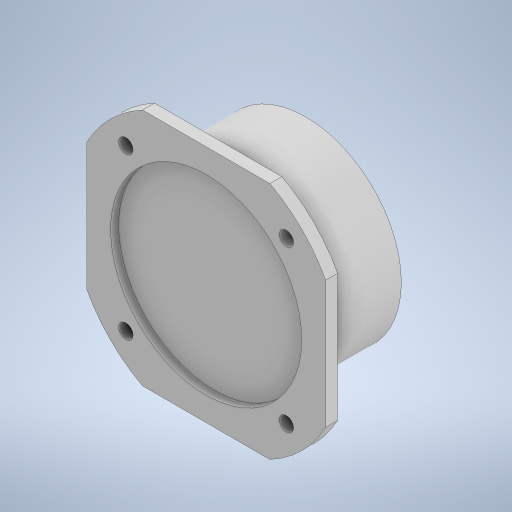
# Autodesk Inventor part: tweetwe
Saved by Autodesk Inventor 2023 (Build 270158000, 158)
## iProperties
Created: 2022-07-14
Part Number: tweetwe
Material: Generic
Document SubType Name: Modeling
Designer: Zain Ali
Density: 1 g/cm^3
Appearance: Default
Author: Zain Ali
Autodesk Inventor part; units mm, degrees
ref_plane "YZ Plane" through (0, 0, 0) normal (1, 0, 0) x (0, 1, 0)
ref_plane "XZ Plane" through (0, 0, 0) normal (0, 1, 0) x (-1, 0, 0)
ref_plane "XY Plane" through (0, 0, 0) normal (0, 0, 1) x (1, 0, 0)
sketch "Sketch1" plane through (0, 0, 0) normal (0, 0, 1) x (1, 0, 0)
  circle A0 centre (0, 0) radius 23.5 construction
  circle A1 centre (0, 0) radius 34 construction
  line L0 (30, 30) -> (-30, 30) construction
  line L1 (-30, 30) -> (-30, -30) construction
  line L2 (-30, -30) -> (30, -30) construction
  line L3 (30, -30) -> (30, 30) construction
  line L4 (30, 30) -> (-30, -30) construction
  line L5 (-30, 30) -> (30, -30) construction
  circle A2 centre (20.1525, 20.1525) radius 4 construction
  circle A3 centre (20.1525, 20.1525) radius 1.8
  arc A4 (30, 16) -> (16, 30) centre (0, 0) ccw
  line L6 (30, 16) -> (30, -16)
  circle A5 centre (0, 0) radius 24
  arc A6 (-16, 30) -> (-30, 16) centre (0, 0) ccw
  line L7 (-16, 30) -> (16, 30)
  circle A7 centre (-20.1525, 20.1525) radius 1.8
  arc A8 (-30, -16) -> (-16, -30) centre (0, 0) ccw
  line L8 (-30, -16) -> (-30, 16)
  circle A9 centre (-20.1525, -20.1525) radius 1.8
  arc A10 (16, -30) -> (30, -16) centre (0, 0) ccw
  line L9 (16, -30) -> (-16, -30)
  circle A11 centre (20.1525, -20.1525) radius 1.8
  line L10 (-35, 35) -> (35, 35)
  line L11 (35, 35) -> (35, -35)
  line L12 (35, -35) -> (-35, -35)
  line L13 (-35, -35) -> (-35, 35)
  line L14 (-35, 35) -> (35, -35) construction
  line L15 (35, 35) -> (-35, -35) construction
  point P0 (-16, -30)
  point P1 (30, -16)
  point P2 (16, 30)
  dimension "d2" = 60
  dimension "d3" = 60
  dimension "d4" = 68
  dimension "d5" = 47
  dimension "d6" = 8
  dimension "d7" = 28.5
  dimension "d8" = 3.6
  dimension "d9" = 48
  dimension "d10" = 360
  dimension "d11" = 70
  dimension "d12" = 70
  constraints: 32 end point, 12 centre point, 12 point on circle, 6 coincident, 4 midpoint, 4 parallel, 4 point on line, 2 horizontal, 2 perpendicular, 1 collinear, 1 concentric, 33 other
  measures "d2" distance of L2.end L4.start
  measures "d3" distance of L2.start L2.end
  measures "d4" diameter of A1
  measures "d5" diameter of A0
  measures "d6" diameter of A2
  measures "d7" distance of A2.centre point (0, 0)
  measures "d8" diameter of A3
  measures "d9" diameter of A5
  measures "d11" distance of L11.start L12.start
  measures "d12" distance of L13.end L11.start
extrude "Extrusion1" add sketch "Sketch1" along normal blind 3 contours L6 A10 L9 A8 L8 A6 L7 A4
extrude "Extrusion2" add sketch "Sketch1" along normal blind 1 contours A5
extrude "Extrusion3" add sketch "Sketch1" against normal blind 22 contours A5
body "Solid1"
